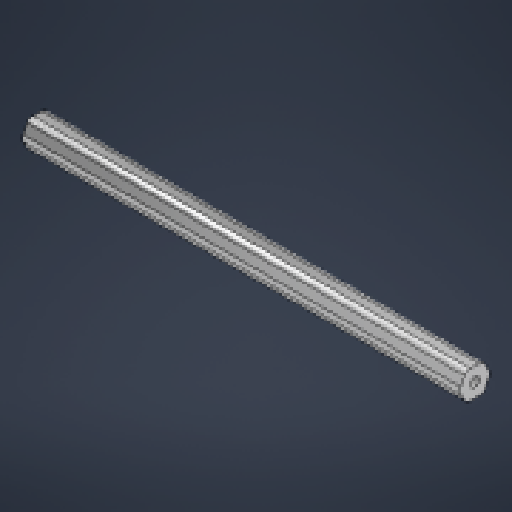
# Autodesk Inventor part: STOCK,HEX,ROUND,HOOD
Saved by Autodesk Inventor 2026.1 (Build 301233020, 233B)
## iProperties
Created: 2026-01-27
Part Number: STOCK,HEX,ROUND,HOOD
Material: Aluminum 6061
Document SubType Name: Modeling
Designer: Owen L
Mass: 76.8632 g
Surface Area: 127.159 cm^2
Volume: 28.4679 cm^3
Density: 2.7 g/cm^3
Appearance: Aluminum - Flat
Author: Owen L
Autodesk Inventor part; units mm, degrees
ref_plane "YZ Plane" through (0, 0, 0) normal (1, 0, 0) x (0, 1, 0)
ref_plane "XZ Plane" through (0, 0, 0) normal (0, 1, 0) x (-1, 0, 0)
ref_plane "XY Plane" through (0, 0, 0) normal (0, 0, 1) x (1, 0, 0)
sketch "Sketch1" plane through (0, 0, 0) normal (1, 0, 0) x (0, 1, 0)
  line L0 (-6.35, -1.9593) -> (-6.35, 1.9593)
  line L1 (-4.8718, 4.5196) -> (-1.4782, 6.4789)
  line L2 (1.4782, 6.4789) -> (4.8718, 4.5196)
  line L3 (6.35, 1.9593) -> (6.35, -1.9593)
  line L4 (4.8718, -4.5196) -> (1.4782, -6.4789)
  line L5 (-1.4782, -6.4789) -> (-4.8718, -4.5196)
  arc A0 (4.8718, -4.5196) -> (6.35, -1.9593) centre (3.3937, -1.9593) ccw
  arc A1 (-1.4782, -6.4789) -> (1.4782, -6.4789) centre (0, -3.9187) ccw
  arc A2 (-6.35, -1.9593) -> (-4.8718, -4.5196) centre (-3.3937, -1.9593) ccw
  arc A3 (-4.8718, 4.5196) -> (-6.35, 1.9593) centre (-3.3937, 1.9593) ccw
  arc A4 (1.4782, 6.4789) -> (-1.4782, 6.4789) centre (0, 3.9187) ccw
  arc A5 (6.35, 1.9593) -> (4.8718, 4.5196) centre (3.3937, 1.9593) ccw
  circle A6 centre (0, 0) radius 6.875 construction
  point P0 (-6.35, -3.6662)
  point P1 (-6.35, 3.6662)
  point P2 (0, 7.3323)
  point P3 (6.35, 3.6662)
  point P4 (6.35, -3.6662)
  point P5 (0, -7.3323)
  dimension "d1" = 12.7
  dimension "d2" = 13.75
  constraints: 13 tangent, 12 end point, 12 point on circle, 12 point on line, 7 centre point, 5 equal radius, 2 coincident, 1 vertical, 13 other
  measures "d1" distance between parallel lines of L0 L3
  measures "d2" diameter of A6
extrude "Extrusion1" add sketch "Sketch1" along normal blind 198.0875
sketch "Sketch2" plane through (0, 0, 0) normal (-1, 0, 0) x (0, 0, 1)
  point P0 (0, 0)
  point P1 (0, 0)
  constraints: 1 coincident
hole "Hole1" at (0, 0, 0) direction (1, 0, 0) diameter 3.9624 end through all thread size "10-32 UNF" class "2B" standard "ANSI Unified Screw Threads"
body "Solid1"
